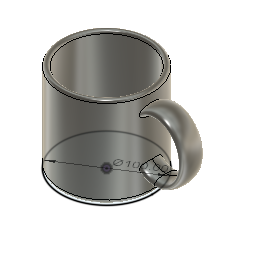
1040김준호_머그컵 (Autodesk Fusion 360 design; units mm, degrees)
Autodesk Fusion 360 part; units mm, degrees
sketch "스케치1" plane through (0, 0, 0) normal (0, 0, 1) x (1, 0, 0)
  circle A0 centre (0, 0) radius 50
  dimension "d1" = 100
  constraint coincident A0.centre origin
  measures "d1" diameter of A0
extrude "돌출1" add sketch "스케치1" along normal blind 100 makes body 1
shell "쉘1" thickness 6 removed faces 1 at (5.3592, -23.4802, 100) on bodies 1
fillet "필렛1" radius 3 2 edges at (-46.6164, -18.0808, 100) (-41.0224, 15.9111, 100) on bodies 1
fillet "필렛2" radius 5 2 edges at (-46.6164, -18.0808, 0) (-41.0224, -15.9111, 6) on bodies 1
sketch "스케치2" plane through (0, 0, 0) normal (0, 1, 0) x (1, 0, 0)
  circle A0 centre (65, -55) radius 32.5
  dimension "d10" = 65
  dimension "d11" = 65
  dimension "d12" = 55
  measures "d10" diameter of A0
  measures "d11" horizontal distance of origin A0.centre
  measures "d12" vertical distance of origin A0.centre
pipe "파이프1" add diameter 10 path "스케치2" along A0 separate body makes body 2
scale "축척1" factors (0.85, 2.5, 1) about (65, 0, 55) bodies 2
extrude "돌출2" cut sketch "스케치1" along normal blind 100 bodies 2
combine "결합1" operation add target body 1 tool bodies 2
equation "main = 100 mm"
equation "d3 = main"
equation "d5 = main * 0.06"
equation "d7 = main * 0.03"
equation "d9 = main * 0.05"
equation "d10 = main * 0.65"
equation "d11 = main * 0.65"
equation "d12 = main * 0.55"
equation "d15 = main * 0.1"
